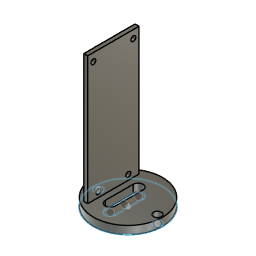
Data Divider Wand Rev A (Autodesk Fusion 360 archive; units mm, degrees)
design "wand hilt 3"
part number: 2025-05-15-15-06-05-558
Autodesk Fusion 360 part; units mm, degrees
sketch "Base" plane through (0, 0, 0) normal (0, 0, 1) x (1, 0, 0)
  circle A0 centre (0, 0) radius 17.5
  circle A1 centre (-15, 0) radius 2
  circle A2 centre (15, 0) radius 2
  line L0 (0.5638, -7.0807) -> (0.5638, 7.0807)
  arc A3 (0.5638, 7.0807) -> (-4.4362, 7.0807) centre (-1.9362, 7.0807) ccw
  line L1 (-4.4362, 7.0807) -> (-4.4362, -7.0807)
  arc A4 (-4.4362, -7.0807) -> (0.5638, -7.0807) centre (-1.9362, -7.0807) ccw
  line L2 (-1.9362, -7.0807) -> (-1.9362, 7.0807) construction
  point P0 (-1.9362, 0)
  dimension "d1" = 35
  dimension "d2" = 4
  dimension "d3" = 4
  dimension "d4" = 15
  dimension "d5" = 15
  dimension "d6" = 5
  constraint tangent L0 A3
  constraint tangent A3 L1
  constraint parallel L0 L1
  constraint tangent L1 A4
  constraint tangent L0 A4
  constraint vertical L2
  constraint midpoint L2 P0
  measures "d1" diameter of A0
  measures "d2" diameter of A1
  measures "d3" diameter of A2
  measures "d4" distance of A0.centre A1.centre
  measures "d5" distance of A0.centre A2.centre
  measures "d6" diameter of A3
extrude "Extrude1" add sketch "Base" along normal blind 4
sketch "Board Bed" plane through (0, 0, 4) normal (0, 0, 1) x (1, 0, 0)
  line L0 (-9.4362, 13) -> (-7.4362, 13)
  line L1 (-7.4362, 13) -> (-7.4362, -13)
  line L2 (-7.4362, -13) -> (-9.4362, -13)
  line L3 (-9.4362, -13) -> (-9.4362, 13)
  circle A0 centre (-15, 0) radius 2
  arc A1 (-4.4362, -7.0807) -> (0.5638, -7.0807) centre (-1.9362, -7.0807) ccw
  line L4 (-4.4362, -7.0807) -> (-4.4362, 7.0807)
  arc A2 (0.5638, 7.0807) -> (-4.4362, 7.0807) centre (-1.9362, 7.0807) ccw
  line L5 (0.5638, 7.0807) -> (0.5638, -7.0807)
  circle A3 centre (15, 0) radius 2
  circle A4 centre (0, 0) radius 17.5
  dimension "d9" = 26
  dimension "d10" = 13
  dimension "d13" = 3
  constraint horizontal L0
  constraint vertical L1
  constraint horizontal L2
  constraint vertical L3
  measures "d9" distance of L0.start L2.end
  measures "d10" distance of L0 A4.centre
  measures "d13" distance of L1 L4
extrude "Extrude2" add sketch "Board Bed" along normal blind 65 contours L0 L1 L2 L3
sketch "Sketch4" plane through (-7.4362, 0, 0) normal (1, 0, 0) x (0, 1, 0)
  line L0 (-13, 4) -> (13, 4)
  line L1 (13, 4) -> (13, 69)
  line L2 (13, 69) -> (-13, 69)
  line L3 (-13, 69) -> (-13, 4)
  circle A0 centre (7.62, 6.58) radius 1.25
  circle A1 centre (-7.62, 6.58) radius 1.25
  circle A2 centre (-10.16, 65) radius 1.25
  circle A3 centre (10.16, 65) radius 1.25
  dimension "d14" = 2.5
  dimension "d15" = 2.5
  dimension "d16" = 15.24
  dimension "d17" = 7.62
  dimension "d18" = 2.5
  dimension "d19" = 2.5
  dimension "d20" = 10.16
  dimension "d21" = 10.16
  dimension "d22" = 20.32
  dimension "d25" = 58.42
  dimension "d26" = 58.42
  dimension "d28" = 2.58
  dimension "d29" = 2.58
  measures "d14" diameter of A0
  measures "d15" diameter of A1
  measures "d16" horizontal distance of A0.centre A1.centre
  measures "d17" horizontal distance of origin A0.centre
  measures "d18" diameter of A2
  measures "d19" diameter of A3
  measures "d20" horizontal distance of origin A2.centre
  measures "d21" horizontal distance of origin A3.centre
  measures "d22" distance of A2.centre A3.centre
  measures "d25" vertical distance of A1.centre A2.centre
  measures "d26" vertical distance of A0.centre A3.centre
  measures "d28" distance of L0 A0.centre
  measures "d29" distance of L0 A1.centre
extrude "Extrude3" cut sketch "Sketch4" against normal blind 5 contours A0 | A1 | A2 | A3

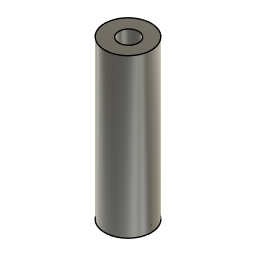
design "wand hilt 2"
part number: 2025-05-15-15-05-41-209
Autodesk Fusion 360 part; units mm, degrees
sketch "Sketch1" plane through (0, 0, 0) normal (0, 0, 1) x (1, 0, 0)
  circle A0 centre (0, 0) radius 17.5
  line L0 (-10, 13) -> (10, 13)
  line L1 (10, 13) -> (10, -13)
  line L2 (10, -13) -> (-10, -13)
  line L3 (-10, -13) -> (-10, 13)
  dimension "d1" = 35
  dimension "d2" = 20
  dimension "d3" = 26
  dimension "d4" = 13
  dimension "d5" = 10
  constraint coincident A0.centre origin
  constraint horizontal L0
  constraint vertical L1
  constraint horizontal L2
  constraint vertical L3
  measures "d1" diameter of A0
  measures "d2" distance of L0.start L0.end
  measures "d3" distance of L0.start L2.end
  measures "d4" distance of A0.centre L0
  measures "d5" distance of A0.centre L1
extrude "Extrude1" add sketch "Sketch1" along normal blind 65
sketch "Sketch2" plane through (0, 0, 65) normal (0, 0, 1) x (-1, 0, 0)
  line L0 (-10, 13) -> (10, 13)
  line L1 (10, 13) -> (10, -13)
  line L2 (10, -13) -> (-10, -13)
  line L3 (-10, -13) -> (-10, 13)
  circle A0 centre (0, 0) radius 17.5
  circle A1 centre (0, 0) radius 17.5
  circle A2 centre (-0.4739, 0) radius 5
  dimension "d8" = 10
  constraint concentric A0 A1
  measures "d8" diameter of A2
extrude "Extrude2" add sketch "Sketch2" along normal blind 2 contours L0 L1 L2 L3 | A0 A1
sketch "Sketch3" plane through (0, 0, 67) normal (0, 0, 1) x (-1, 0, 0)
  circle A0 centre (-0.4739, 0) radius 5
  circle A1 centre (0, 0) radius 17.5
  circle A2 centre (-0.4739, 0) radius 7.5
  dimension "d11" = 15
  constraint concentric A0 A2
  measures "d11" diameter of A2
extrude "Extrude3" add sketch "Sketch3" along normal blind 52 contours A1
fillet "Fillet1" radius 3 1 edges at (7.4663, 2.7121, 67)
form "Form1" [no effect]
sketch "Sketch4" plane through (0, 0, 0) normal (0, 0, 1) x (1, 0, 0)
  circle A0 centre (-15, 0) radius 2
  circle A1 centre (0, 0) radius 17.5
  circle A2 centre (15, 0) radius 2
  dimension "d16" = 4
  dimension "d17" = 15
  dimension "d18" = 4
  dimension "d19" = 15
  measures "d16" diameter of A0
  measures "d17" distance of A0.centre A1.centre
  measures "d18" diameter of A2
  measures "d19" distance of A2.centre A1.centre
extrude "Extrude4" cut sketch "Sketch4" along normal blind 5 contours A0 | A2
